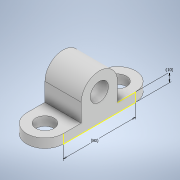
# Autodesk Inventor part: Tarea 1 Dinamica Lab
Saved by Autodesk Inventor 2022 (Build 260153000, 153)
## iProperties
Created: 2024-01-24
Part Number: Tarea 1 Dinamica Lab
Material: Generic
Document SubType Name: Modeling
Designer: HP15BW010LA
Density: 1 g/cm^3
Appearance: Default
Author: HP15BW010LA
Autodesk Inventor part; units mm, degrees
ref_plane "YZ Plane" through (0, 0, 0) normal (1, 0, 0) x (0, 1, 0)
ref_plane "XZ Plane" through (0, 0, 0) normal (0, 1, 0) x (-1, 0, 0)
ref_plane "XY Plane" through (0, 0, 0) normal (0, 0, 1) x (1, 0, 0)
sketch "Sketch1" plane through (0, 0, 0) normal (0, 1, 0) x (-1, 0, 0)
  line L0 (-20, 20) -> (-20, -20)
  line L1 (20, -20) -> (20, 20)
  line L2 (20, 20) -> (-20, -20) construction
  line L3 (-20, 20) -> (20, -20) construction
  line L4 (0, 20) -> (0, 40) construction
  circle A0 centre (0, 40) radius 10
  arc A1 (20, 40) -> (-20, 40) centre (0, 40) ccw
  line L5 (0, -20) -> (0, -40) construction
  circle A2 centre (0, -40) radius 10
  arc A3 (-20, -40) -> (20, -40) centre (0, -40) ccw
  line L6 (20, 20) -> (20, 40)
  line L7 (20, -20) -> (20, -40)
  line L8 (-20, -20) -> (-20, -40)
  line L9 (-20, 20) -> (-20, 40)
  point P0 (0, 0)
  dimension "d3" = 20
  dimension "d6" = 20
  constraints: 20 end point, 4 centre point, 4 coincident, 4 point on circle, 2 midpoint, 2 parallel, 2 point on line, 2 vertical, 1 tangent
  measures "d3" diameter of A0
  measures "d6" diameter of A2
extrude "Extrusion1" add sketch "Sketch1" along normal blind 10
sketch "Sketch2" plane through (20, 0, 40) normal (1, 0, 0) x (0, 0, -1)
  line L0 (80, 10) -> (0, 10) projected
  line L1 (40, 10) -> (40, 30)
  arc A0 (60, 30) -> (20, 30) centre (40, 30) ccw
  circle A1 centre (40, 30) radius 10
  line L2 (20, 30) -> (20, 10)
  line L3 (60, 30) -> (60, 10)
  line L4 (20, 10) -> (60, 10)
  line L5 (0, 10) -> (80, 10) projected
  point P0 (40, 0)
  dimension "d11" = 40
  dimension "d12" = 20
  constraints: 8 end point, 3 tangent, 2 centre point, 2 coincident, 2 midpoint, 2 perpendicular, 2 point on circle, 2 point on line, 1 collinear, 1 vertical
  measures "d11" diameter of A0
  measures "d12" diameter of A1
extrude "Extrusion2" add sketch "Sketch2" against normal blind 40
sketch "Sketch3" plane through (20, 0, 40) normal (1, 0, 0) x (0, 0, -1)
  line L0 (80, 0) -> (80, 10) projected
  line L1 (0, 0) -> (0, 10) projected
  line L2 (60, 10) -> (80, 10) projected
  line L3 (0, 0) -> (80, 0) projected
  point P0 (40, 0)
  dimension "d15" = 80
  dimension "d16" = 10
  measures "d15" distance between parallel lines of L0 L1
  measures "d16" distance between parallel lines of L2 L3
body "Solid1"
